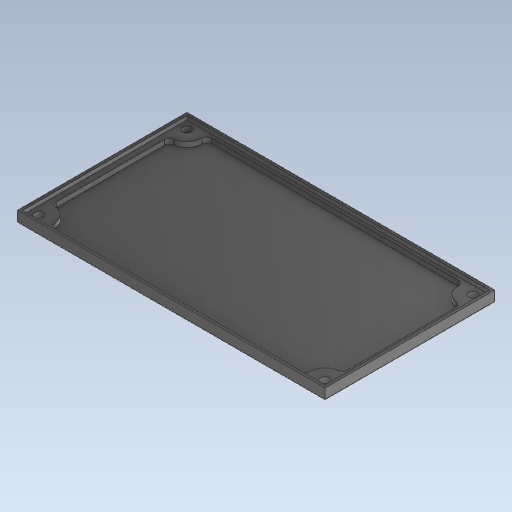
# Autodesk Inventor part: MainBoard_cover
Saved by Autodesk Inventor 2020 (Build 240168000, 168)
## iProperties
Part Number: MainBoard_cover
Material: 一般
Document SubType Name: Modeling
Designer: Masato Kubotera
Density: 1 g/cm^3
Appearance: 滑らか - 黒
Description: PLA
Mass: 6.13737 g
Surface Area: 193.634 cm^2
Volume: 6.13737 cm^3
Author: Masato Kubotera
Autodesk Inventor part; units mm, degrees
ref_plane "YZ Plane" through (0, 0, 0) normal (1, 0, 0) x (0, 1, 0)
ref_plane "XZ Plane" through (0, 0, 0) normal (0, 1, 0) x (-1, 0, 0)
ref_plane "XY Plane" through (0, 0, 0) normal (0, 0, 1) x (1, 0, 0)
derived "MainBoard.ipt"
sketch "スケッチ3" plane through (0, 0, -88.5) normal (0, 0, 1) x (1, 0, 0)
  line L0 (20.25, -135) -> (20.25, 0)
  line L1 (-80.25, 0) -> (-80.25, -135)
  line L2 (-30, -135) -> (-30, 0) construction
  line L3 (-80.25, -67.5) -> (20.25, -67.5) construction
  line L4 (-55, 1.4849) -> (-55, 5)
  line L5 (-55, 5) -> (-5, 5)
  line L6 (-5, 5) -> (-5, 1.4849)
  arc A0 (-56.4849, 0) -> (-55, 1.4849) centre (-55.7425, 0.7425) ccw
  arc A1 (-5, 1.4849) -> (-3.5151, 0) centre (-4.2575, 0.7425) ccw
  line L7 (-56.4849, 0) -> (-80.25, 0)
  line L8 (20.25, 0) -> (-3.5151, 0)
  line L9 (-5, 0) -> (-55, 0)
  line L10 (-55, -136.4849) -> (-55, -140)
  line L11 (-55, -140) -> (-5, -140)
  line L12 (-5, -140) -> (-5, -136.4849)
  arc A2 (-55, -136.4849) -> (-56.4849, -135) centre (-55.7425, -135.7425) ccw
  arc A3 (-3.5151, -135) -> (-5, -136.4849) centre (-4.2575, -135.7425) ccw
  line L13 (-56.4849, -135) -> (-80.25, -135)
  line L14 (20.25, -135) -> (-3.5151, -135)
  line L15 (-5, -135) -> (-55, -135)
  line L16 (18, -127.5) -> (-47, -127.5) construction
  line L17 (-47, -127.5) -> (-47, -7.5) construction
  line L18 (-47, -7.5) -> (18, -7.5) construction
  line L19 (18, -7.5) -> (18, -127.5) construction
  line L20 (18, -127.5) -> (-47, -7.5) construction
  line L21 (-47, -127.5) -> (18, -7.5) construction
  line L22 (-46, -116.5) -> (-46, -18.5)
  line L23 (-36.0627, -9.5) -> (7.0627, -9.5)
  line L24 (15, -10.5) -> (-44, -10.5) construction
  line L25 (-44, -10.5) -> (-44, -124.5) construction
  line L26 (-44, -124.5) -> (15, -124.5) construction
  line L27 (15, -124.5) -> (15, -10.5) construction
  line L28 (15, -10.5) -> (-44, -124.5) construction
  line L29 (-44, -10.5) -> (15, -124.5) construction
  circle A4 centre (15, -10.5) radius 2
  circle A5 centre (-44, -10.5) radius 2
  arc A6 (-44, -16.5) -> (-38.0471, -11.25) centre (-44, -10.5) ccw
  arc A7 (9.0471, -11.25) -> (15, -16.5) centre (15, -10.5) ccw
  line L30 (17, -18.5) -> (17, -116.5)
  line L31 (-14.5, -7.5) -> (-14.5, -127.5) construction
  line L32 (-73.25, -65) -> (-54, -65)
  line L33 (-52, -63) -> (-52, -7)
  line L34 (-54, -5) -> (-73.25, -5)
  line L35 (-75.25, -7) -> (-75.25, -63)
  arc A8 (-75.25, -63) -> (-73.25, -65) centre (-73.25, -63) ccw
  arc A9 (-54, -65) -> (-52, -63) centre (-54, -63) ccw
  arc A10 (-52, -7) -> (-54, -5) centre (-54, -7) ccw
  arc A11 (-73.25, -5) -> (-75.25, -7) centre (-73.25, -7) ccw
  arc A12 (-44, -16.5) -> (-46, -18.5) centre (-44, -18.5) ccw
  arc A13 (-36.0627, -9.5) -> (-38.0471, -11.25) centre (-36.0627, -11.5) ccw
  arc A14 (9.0471, -11.25) -> (7.0627, -9.5) centre (7.0627, -11.5) ccw
  arc A15 (17, -18.5) -> (15, -16.5) centre (15, -18.5) ccw
  line L36 (-36.0627, -125.5) -> (7.0627, -125.5)
  circle A16 centre (15, -124.5) radius 2
  circle A17 centre (-44, -124.5) radius 2
  arc A18 (-38.0471, -123.75) -> (-44, -118.5) centre (-44, -124.5) ccw
  arc A19 (15, -118.5) -> (9.0471, -123.75) centre (15, -124.5) ccw
  line L37 (-73.25, -70) -> (-54, -70)
  line L38 (-52, -72) -> (-52, -128)
  line L39 (-54, -130) -> (-73.25, -130)
  line L40 (-75.25, -128) -> (-75.25, -72)
  arc A20 (-73.25, -70) -> (-75.25, -72) centre (-73.25, -72) ccw
  arc A21 (-52, -72) -> (-54, -70) centre (-54, -72) ccw
  arc A22 (-54, -130) -> (-52, -128) centre (-54, -128) ccw
  arc A23 (-75.25, -128) -> (-73.25, -130) centre (-73.25, -128) ccw
  arc A24 (-46, -116.5) -> (-44, -118.5) centre (-44, -116.5) ccw
  arc A25 (-38.0471, -123.75) -> (-36.0627, -125.5) centre (-36.0627, -123.5) ccw
  arc A26 (7.0627, -125.5) -> (9.0471, -123.75) centre (7.0627, -123.5) ccw
  arc A27 (15, -118.5) -> (17, -116.5) centre (15, -116.5) ccw
  point P0 (0, 0)
  point P1 (-30, -67.5)
  point P2 (-55, 0)
  point P3 (-14.5, -67.5)
  point P4 (-46, -16.1569)
  point P5 (-38.0839, -9.5)
  point P6 (9.0839, -9.5)
  point P7 (17, -16.1569)
ref_plane "作業平面1" through (20.25, 0, -88.5) normal (0, 0, -1) x (0, -1, 0)
sketch "スケッチ4" plane through (20.25, 0, -88.5) normal (0, 0, -1) x (0, -1, 0)
  line L0 (6.25, 68.5) -> (128.75, 68.5)
  line L1 (128.75, 68.5) -> (128.75, 1)
  line L2 (128.75, 1) -> (6.25, 1)
  line L3 (6.25, 1) -> (6.25, 68.5)
  line L4 (6.25, 68.5) -> (128.75, 1) construction
  line L5 (128.75, 68.5) -> (6.25, 1) construction
  line L6 (7.25, 67.5) -> (127.75, 67.5)
  line L7 (127.75, 67.5) -> (127.75, 2)
  line L8 (127.75, 2) -> (7.25, 2)
  line L9 (7.25, 2) -> (7.25, 67.5)
  line L10 (7.25, 67.5) -> (127.75, 2) construction
  line L11 (127.75, 67.5) -> (7.25, 2) construction
  line L12 (7.5, 2.25) -> (127.5, 2.25) construction
  line L13 (7.5, 67.25) -> (7.5, 2.25) construction
  circle A0 centre (10.5, 5.25) radius 1.75
  circle A1 centre (10.5, 64.25) radius 1.75
  circle A2 centre (124.5, 5.25) radius 1.75
  circle A3 centre (124.5, 64.25) radius 1.75
  line L14 (9.5, 56.3127) -> (9.5, 13.1873) projected
  arc A4 (9.5, 13.1873) -> (11.25, 11.2029) centre (11.5, 13.1873) ccw projected
  arc A5 (16.5, 5.25) -> (11.25, 11.2029) centre (10.5, 5.25) ccw projected
  arc A6 (16.5, 5.25) -> (18.5, 3.25) centre (18.5, 5.25) ccw projected
  arc A7 (11.25, 58.2971) -> (9.5, 56.3127) centre (11.5, 56.3127) ccw projected
  arc A8 (11.25, 58.2971) -> (16.5, 64.25) centre (10.5, 64.25) ccw projected
  arc A9 (18.5, 66.25) -> (16.5, 64.25) centre (18.5, 64.25) ccw projected
  line L15 (116.5, 66.25) -> (18.5, 66.25) projected
  arc A10 (118.5, 64.25) -> (116.5, 66.25) centre (116.5, 64.25) ccw projected
  arc A11 (118.5, 64.25) -> (123.75, 58.2971) centre (124.5, 64.25) ccw projected
  arc A12 (125.5, 56.3127) -> (123.75, 58.2971) centre (123.5, 56.3127) ccw projected
  line L16 (125.5, 56.3127) -> (125.5, 13.1873) projected
  arc A13 (123.75, 11.2029) -> (125.5, 13.1873) centre (123.5, 13.1873) ccw projected
  arc A14 (123.75, 11.2029) -> (118.5, 5.25) centre (124.5, 5.25) ccw projected
  arc A15 (116.5, 3.25) -> (118.5, 5.25) centre (116.5, 5.25) ccw projected
  line L17 (18.5, 3.25) -> (116.5, 3.25) projected
  point P0 (0, 20.25)
  point P1 (67.5, 34.75)
  point P2 (67.5, 34.75)
  point P3 (67.5, 34.75)
  point P4 (67.5, 34.75)
  dimension "d5" = 1
  dimension "d6" = 1
  dimension "d7" = 0.25
  dimension "d8" = 0.25
  dimension "d11" = 3.5
  dimension "d12" = 3.5
  dimension "d13" = 3.5
  dimension "d14" = 3.5
  constraints: 24 end point, 6 midpoint, 5 coincident, 4 centre point, 4 parallel, 2 horizontal, 2 perpendicular
  measures "d5" distance between parallel lines of L2 L8
  measures "d6" distance between parallel lines of L3 L9
  measures "d7" distance between parallel lines of L8 L12
  measures "d8" distance between parallel lines of L13 L9
  measures "d11" diameter of A0
  measures "d12" diameter of A1
  measures "d13" diameter of A2
  measures "d14" diameter of A3
extrude "押し出し1" add sketch "スケッチ4" against normal blind 4 contours L0 L1 L2 L3
extrude "押し出し2" add sketch "スケッチ4" against normal blind 2.4 contours L6 L7 L8 L9
extrude "押し出し3" add sketch "スケッチ3" along normal blind 0.4 contours L22 A12 A6 A13 L23 A14 A7 A15 L30 A27 A19 A26 L36 A25 A18 A24
equation "\"d6\" = d5"
equation "\"d8\" = d7"
equation "\"d12\" = d11"
equation "\"d13\" = d11"
equation "\"d14\" = d11"
